Autodesk Fusion 360 part; units mm, degrees
(part 2 of 2)
sketch "Sketch12" plane through (62, 0, 0) normal (1, 0, 0) x (0, 1, 0)
  circle A0 centre (-85.8, 13) radius 2
  circle A1 centre (74.2, 31) radius 2
  circle A2 centre (-85.8, 31) radius 2
  circle A3 centre (74.2, 13) radius 2
  line L0 (-112.5, 0) -> (112.5, 0)
  line L1 (112.5, 0) -> (112.5, 41)
  line L2 (112.5, 41) -> (-112.5, 41)
  line L3 (-112.5, 41) -> (-112.5, 0)
  line L4 (-93.5, 20.2) -> (-91, 20.2)
  line L5 (-91, 20.2) -> (-91, 13.3)
  line L6 (-91, 13.3) -> (-93.5, 13.3)
  line L7 (-93.5, 13.3) -> (-93.5, 20.2)
  line L8 (-81.4787, 20.2) -> (-78.9787, 20.2)
  line L9 (-78.9787, 20.2) -> (-78.9787, 13.3)
  line L10 (-78.9787, 13.3) -> (-81.4787, 13.3)
  line L11 (-81.4787, 13.3) -> (-81.4787, 20.2)
  line L12 (-85.8, 13) -> (-85.8, 31) construction
  line L13 (74.2, 31) -> (74.2, 13) construction
  line L14 (81.9, 20.2) -> (81.9, 13.3)
  line L15 (79.4, 13.3) -> (79.4, 20.2)
  line L16 (69, 20.2) -> (69, 13.3)
  line L17 (79.4, 20.2) -> (81.9, 20.2)
  line L18 (69, 13.3) -> (66.5, 13.3)
  line L19 (81.9, 13.3) -> (79.4, 13.3)
  line L20 (66.5, 13.3) -> (66.5, 20.2)
  line L21 (66.5, 20.2) -> (69, 20.2)
  point P0 (73.9672, 16.2288)
  point P1 (73.9672, 16.2288)
  dimension "d89" = 2.5
  dimension "d90" = 6.9
  dimension "d91" = 5.2
  dimension "d92" = 4.3213
  dimension "d93" = 13.3
  dimension "d94" = 2.5
  dimension "d95" = 6.9
  dimension "d96" = 5.2
  dimension "d97" = 13.3
  dimension "d98" = 5.2
  constraint horizontal L4
  constraint vertical L5
  constraint horizontal L6
  constraint vertical L7
  constraint horizontal L8
  constraint vertical L9
  constraint horizontal L10
  constraint vertical L11
  constraint equal L4 L8
  constraint equal L7 L11
  constraint collinear L4 L8
  constraint coincident A0.centre L12.start
  constraint coincident A2.centre L12.end
  constraint coincident A1.centre L13.start
  constraint coincident A3.centre L13.end
  constraint horizontal L21
  constraint vertical L16
  constraint horizontal L18
  constraint vertical L20
  constraint horizontal L17
  constraint vertical L14
  constraint horizontal L19
  constraint vertical L15
  constraint equal L17 L21
  constraint equal L15 L20
  constraint collinear L17 L21
  constraint coincident P1 P0
  measures "d89" distance of L5.end L6.end
  measures "d90" distance of L4.start L6.end
  measures "d91" distance of L5 L12
  measures "d92" distance of L11 L12
  measures "d93" distance of L0 L6
  measures "d94" distance of L18.end L16.end
  measures "d95" distance of L20.end L18.end
  measures "d96" distance of L13 L16
  measures "d97" distance of L0 L18
  measures "d98" distance of L13 L15
extrude "Extrude13" cut sketch "Sketch12" against normal through all contours L4 L5 L6 L7 | L8 L9 L10 L11 | L14 L15 L17 L19 | L16 L18 L20 L21 bodies 1
sketch "Sketch13" plane through (62, 0, 0) normal (1, 0, 0) x (0, 1, 0)
  line L0 (66.5, 20.2) -> (69, 20.2)
  line L1 (69, 20.2) -> (69, 13.3)
  line L2 (69, 13.3) -> (66.5, 13.3)
  line L3 (66.5, 13.3) -> (66.5, 20.2)
  line L4 (-93.5, 13.3) -> (-93.5, 20.2)
  line L5 (-93.5, 20.2) -> (-91, 20.2)
  line L6 (-91, 20.2) -> (-91, 13.3)
  line L7 (-91, 13.3) -> (-93.5, 13.3)
  line L8 (81.9, 13.3) -> (79.4, 13.3)
  line L9 (79.4, 13.3) -> (79.4, 20.2)
  line L10 (79.4, 20.2) -> (81.9, 20.2)
  line L11 (81.9, 20.2) -> (81.9, 13.3)
  line L12 (-81.4787, 13.3) -> (-81.4787, 20.2)
  line L13 (-81.4787, 20.2) -> (-78.9787, 20.2)
  line L14 (-78.9787, 20.2) -> (-78.9787, 13.3)
  line L15 (-78.9787, 13.3) -> (-81.4787, 13.3)
  circle A0 centre (-85.8, 13) radius 2
  circle A1 centre (74.2, 31) radius 2
  circle A2 centre (-85.8, 31) radius 2
  circle A3 centre (74.2, 13) radius 2
  line L16 (-112.5, 0) -> (112.5, 0)
  line L17 (112.5, 0) -> (112.5, 41)
  line L18 (112.5, 41) -> (-112.5, 41)
  line L19 (-112.5, 41) -> (-112.5, 0)
  line L20 (47, 17.6) -> (62, 17.6)
  line L21 (62, 17.6) -> (62, 8.6)
  line L22 (62, 8.6) -> (47, 8.6)
  line L23 (47, 8.6) -> (47, 17.6)
  dimension "d100" = 15
  dimension "d101" = 9
  dimension "d102" = 8.6
  dimension "d103" = 50.5
  constraint horizontal L20
  constraint vertical L21
  constraint horizontal L22
  constraint vertical L23
  measures "d100" distance of L20.start L20.end
  measures "d101" distance of L20.start L22.end
  measures "d102" distance of L16 L22
  measures "d103" distance of L17 L21
extrude "Extrude14" cut sketch "Sketch13" against normal blind 2 contours L20 L21 L22 L23 bodies 1
sketch "Sketch14" plane through (62, 0, 0) normal (1, 0, 0) x (0, 1, 0)
  line L0 (62, 17.6) -> (62, 8.6)
  line L1 (62, 8.6) -> (47, 8.6)
  line L2 (47, 8.6) -> (47, 17.6)
  line L3 (47, 17.6) -> (62, 17.6)
  line L4 (66.5, 20.2) -> (69, 20.2)
  line L5 (69, 20.2) -> (69, 13.3)
  line L6 (69, 13.3) -> (66.5, 13.3)
  line L7 (66.5, 13.3) -> (66.5, 20.2)
  line L8 (-93.5, 13.3) -> (-93.5, 20.2)
  line L9 (-93.5, 20.2) -> (-91, 20.2)
  line L10 (-91, 20.2) -> (-91, 13.3)
  line L11 (-91, 13.3) -> (-93.5, 13.3)
  line L12 (81.9, 13.3) -> (79.4, 13.3)
  line L13 (79.4, 13.3) -> (79.4, 20.2)
  line L14 (79.4, 20.2) -> (81.9, 20.2)
  line L15 (81.9, 20.2) -> (81.9, 13.3)
  line L16 (-81.4787, 13.3) -> (-81.4787, 20.2)
  line L17 (-81.4787, 20.2) -> (-78.9787, 20.2)
  line L18 (-78.9787, 20.2) -> (-78.9787, 13.3)
  line L19 (-78.9787, 13.3) -> (-81.4787, 13.3)
  circle A0 centre (-85.8, 13) radius 2
  circle A1 centre (74.2, 31) radius 2
  circle A2 centre (-85.8, 31) radius 2
  circle A3 centre (74.2, 13) radius 2
  line L20 (-112.5, 0) -> (112.5, 0)
  line L21 (112.5, 0) -> (112.5, 41)
  line L22 (112.5, 41) -> (-112.5, 41)
  line L23 (-112.5, 41) -> (-112.5, 0)
  line L24 (-112.5, 5) -> (110.5, 5)
  line L25 (43.4, 5) -> (43.4, 21.2)
  line L26 (43.4, 21.2) -> (65.6, 21.2)
  line L27 (65.6, 21.2) -> (65.6, 5)
  line L28 (65.6, 5) -> (43.4, 5)
  dimension "d106" = -3.6
extrude "Extrude15" add sketch "Sketch14" against normal blind 7 from surface at -5 separate body contours L24 L25 L26 L27 L28 makes body 4
extrude "Extrude16" add sketch "Sketch14" along normal blind 6.9 from surface at -12 contours L0 L1 L2 L3 bodies 4
extrude "Extrude17" cut 1 faces at (54.6667, 50.8, 5) along direction (0, 0, 1) blind 1.7 on bodies 4 bodies 4
sketch "Sketch15" plane through (0, 0, 39) normal (0, 0, -1) x (1, 0, 0)
  line L0 (-42.3, 34.3) -> (-12.3, 34.3)
  arc A0 (-12.3, 29.3) -> (-12.3, 34.3) centre (-12.3, 31.8) ccw
  line L1 (-12.3, 29.3) -> (-42.3, 29.3)
  arc A1 (-42.3, 34.3) -> (-42.3, 29.3) centre (-42.3, 31.8) ccw
  line L2 (-42.3, 44.3) -> (-12.3, 44.3)
  arc A2 (-12.3, 39.3) -> (-12.3, 44.3) centre (-12.3, 41.8) ccw
  line L3 (-12.3, 39.3) -> (-42.3, 39.3)
  arc A3 (-42.3, 44.3) -> (-42.3, 39.3) centre (-42.3, 41.8) ccw
  line L4 (-42.3, 24.3) -> (-12.3, 24.3)
  arc A4 (-12.3, 19.3) -> (-12.3, 24.3) centre (-12.3, 21.8) ccw
  line L5 (-12.3, 19.3) -> (-42.3, 19.3)
  arc A5 (-42.3, 24.3) -> (-42.3, 19.3) centre (-42.3, 21.8) ccw
  line L6 (-42.3, 74.3) -> (-12.3, 74.3)
  arc A6 (-12.3, 69.3) -> (-12.3, 74.3) centre (-12.3, 71.8) ccw
  line L7 (-12.3, 69.3) -> (-42.3, 69.3)
  arc A7 (-42.3, 74.3) -> (-42.3, 69.3) centre (-42.3, 71.8) ccw
  line L8 (45.7, 29.3) -> (15.7, 29.3)
  arc A8 (15.7, 34.3) -> (15.7, 29.3) centre (15.7, 31.8) ccw
  line L9 (15.7, 34.3) -> (45.7, 34.3)
  arc A9 (45.7, 29.3) -> (45.7, 34.3) centre (45.7, 31.8) ccw
  circle A10 centre (-29, -58) radius 2
  circle A11 centre (-29, -67) radius 2
  circle A12 centre (-20, -58) radius 2
  circle A13 centre (-20, -67) radius 2
  arc A14 (-34.5896, -90.2209) -> (-14.4104, -90.2209) centre (-24.5, -62.5) ccw
  arc A15 (-32.5375, -84.5828) -> (-34.5896, -90.2209) centre (-33.5635, -87.4019) ccw
  arc A16 (-32.5375, -84.5828) -> (-16.4625, -84.5828) centre (-24.5, -62.5) ccw
  arc A17 (-14.4104, -90.2209) -> (-16.4625, -84.5828) centre (-15.4365, -87.4019) ccw
  arc A18 (-9.2972, -47.2972) -> (-18.9354, -41.7326) centre (-24.5, -62.5) ccw
  arc A19 (-13.5398, -51.5398) -> (-9.2972, -47.2972) centre (-11.4185, -49.4185) ccw
  arc A20 (-13.5398, -51.5398) -> (-20.4883, -47.5281) centre (-24.5, -62.5) ccw
  arc A21 (-18.9354, -41.7326) -> (-20.4883, -47.5281) centre (-19.7118, -44.6304) ccw
  arc A22 (-45.2674, -56.9354) -> (-45.2674, -68.0646) centre (-24.5, -62.5) ccw
  arc A23 (-39.4719, -58.4883) -> (-45.2674, -56.9354) centre (-42.3696, -57.7118) ccw
  arc A24 (-39.4719, -58.4883) -> (-39.4719, -66.5117) centre (-24.5, -62.5) ccw
  arc A25 (-45.2674, -68.0646) -> (-39.4719, -66.5117) centre (-42.3696, -67.2882) ccw
  arc A26 (-39.7028, -77.7028) -> (-30.0646, -83.2674) centre (-24.5, -62.5) ccw
  arc A27 (-35.4602, -73.4602) -> (-39.7028, -77.7028) centre (-37.5815, -75.5815) ccw
  arc A28 (-35.4602, -73.4602) -> (-28.5117, -77.4719) centre (-24.5, -62.5) ccw
  arc A29 (-30.0646, -83.2674) -> (-28.5117, -77.4719) centre (-29.2882, -80.3696) ccw
  arc A30 (-14.4104, -34.7791) -> (-34.5896, -34.7791) centre (-24.5, -62.5) ccw
  arc A31 (-16.4625, -40.4172) -> (-14.4104, -34.7791) centre (-15.4365, -37.5981) ccw
  arc A32 (-16.4625, -40.4172) -> (-32.5375, -40.4172) centre (-24.5, -62.5) ccw
  arc A33 (-34.5896, -34.7791) -> (-32.5375, -40.4172) centre (-33.5635, -37.5981) ccw
  arc A34 (-53.5518, -67.6226) -> (-43.4622, -85.0983) centre (-24.5, -62.5) ccw
  arc A35 (-47.643, -66.5807) -> (-53.5518, -67.6226) centre (-50.5974, -67.1017) ccw
  arc A36 (-47.643, -66.5807) -> (-39.6055, -80.502) centre (-24.5, -62.5) ccw
  arc A37 (-43.4622, -85.0983) -> (-39.6055, -80.502) centre (-41.5339, -82.8002) ccw
  arc A38 (-5.5378, -85.0983) -> (4.5518, -67.6226) centre (-24.5, -62.5) ccw
  arc A39 (-9.3945, -80.502) -> (-5.5378, -85.0983) centre (-7.4661, -82.8002) ccw
  arc A40 (-9.3945, -80.502) -> (-1.357, -66.5807) centre (-24.5, -62.5) ccw
  arc A41 (4.5518, -67.6226) -> (-1.357, -66.5807) centre (1.5974, -67.1017) ccw
  arc A42 (-3.7326, -68.0646) -> (-3.7326, -56.9354) centre (-24.5, -62.5) ccw
  arc A43 (-9.5281, -66.5117) -> (-3.7326, -68.0646) centre (-6.6304, -67.2882) ccw
  arc A44 (-9.5281, -66.5117) -> (-9.5281, -58.4883) centre (-24.5, -62.5) ccw
  arc A45 (-3.7326, -56.9354) -> (-9.5281, -58.4883) centre (-6.6304, -57.7118) ccw
  arc A46 (-30.0646, -41.7326) -> (-39.7028, -47.2972) centre (-24.5, -62.5) ccw
  arc A47 (-28.5117, -47.5281) -> (-30.0646, -41.7326) centre (-29.2882, -44.6304) ccw
  arc A48 (-28.5117, -47.5281) -> (-35.4602, -51.5398) centre (-24.5, -62.5) ccw
  arc A49 (-39.7028, -47.2972) -> (-35.4602, -51.5398) centre (-37.5815, -49.4185) ccw
  arc A50 (-18.9354, -83.2674) -> (-9.2972, -77.7028) centre (-24.5, -62.5) ccw
  arc A51 (-20.4883, -77.4719) -> (-18.9354, -83.2674) centre (-19.7118, -80.3696) ccw
  arc A52 (-20.4883, -77.4719) -> (-13.5398, -73.4602) centre (-24.5, -62.5) ccw
  arc A53 (-9.2972, -77.7028) -> (-13.5398, -73.4602) centre (-11.4185, -75.5815) ccw
  arc A54 (4.5518, -57.3774) -> (-5.5378, -39.9017) centre (-24.5, -62.5) ccw
  arc A55 (-1.357, -58.4193) -> (4.5518, -57.3774) centre (1.5974, -57.8983) ccw
  arc A56 (-1.357, -58.4193) -> (-9.3945, -44.498) centre (-24.5, -62.5) ccw
  arc A57 (-5.5378, -39.9017) -> (-9.3945, -44.498) centre (-7.4661, -42.1998) ccw
  arc A58 (-43.4622, -39.9017) -> (-53.5518, -57.3774) centre (-24.5, -62.5) ccw
  arc A59 (-39.6055, -44.498) -> (-43.4622, -39.9017) centre (-41.5339, -42.1998) ccw
  arc A60 (-39.6055, -44.498) -> (-47.643, -58.4193) centre (-24.5, -62.5) ccw
  arc A61 (-53.5518, -57.3774) -> (-47.643, -58.4193) centre (-50.5974, -57.8983) ccw
  line L10 (60, 96.1) -> (-60, 96.1)
  line L11 (-60, 96.1) -> (-60, -110.5)
  line L12 (-60, -110.5) -> (60, -110.5)
  line L13 (60, -110.5) -> (60, 96.1)
  line L14 (60, 96.1) -> (-60, 96.1)
  line L15 (60, 94.1) -> (-60, 94.1)
  dimension "d115" = -2
extrude "Extrude18" add sketch "Sketch15" along normal blind 16.5 contours L10 L11 L13 L14 L15 bodies 1
equation "d38 = ( 3 / 2 ) * 1 mm + 4 mm"
equation "d39 = ( 7 / 2 ) * 1 mm + 3 mm"
equation "d40 = ( 7 / 2 ) * 1 mm + 12.5 mm"
equation "d62 = ( 360 / 18 / 2 ) * 1 deg"
equation "d72 = 35 mm - 5 mm"
equation "d85 = -23 mm - 35 mm"
equation "d116 = 18.5 mm - 2 mm"
